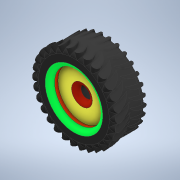
# Autodesk Inventor part: wheel 2
Saved by Autodesk Inventor 2021.3 (Build 253353000, 353)
## iProperties
Created: 2021-07-27
Part Number: wheel 2
Material: Rubber
Document SubType Name: Modeling
Designer: ASUS
Density: 0.93 g/cm^3
Appearance: Rubber - Black
Author: ASUS
Autodesk Inventor part; units mm, degrees
ref_plane "YZ Plane" through (0, 0, 0) normal (1, 0, 0) x (0, 1, 0)
ref_plane "XY Plane" through (0, 0, 0) normal (0, 0, 1) x (1, 0, 0)
sketch "Sketch1" plane through (0, 0, 0) normal (0, 0, 1) x (1, 0, 0)
  circle A0 centre (0, 0) radius 25
  dimension "d0" = 50
  constraints: 1 centre point, 1 coincident
  measures "d0" diameter of A0
extrude "Extrusion1" add sketch "Sketch1" along normal blind 20
fillet "Fillet1" radius 3 2 edges at (-25, 0, 20) (-25, 0, 0)
ref_plane "Work Plane1" through (0, 25, 0) normal (0, 1, 0) x (-1, 0, 0)
sketch "Sketch3" plane through (0, 25, 0) normal (0, 1, 0) x (-1, 0, 0)
  line L0 (25, 3) -> (25, 17) projected
  line L1 (25, 10) -> (-25, 10)
  line L2 (-25, 3) -> (-25, 17) projected
  line L3 (22, 0) -> (-22, 0) projected
  arc A0 (0, 10) -> (-1.7253, 1.0245) centre (24.2725, 0.6808) ccw
  arc A1 (0, 10) -> (-3.7943, 0.9149) centre (6.1349, 2.103) ccw
  arc A2 (-3.7943, 0.9149) -> (-1.7253, 1.0245) centre (-2.7634, 1.0382) ccw
  line L4 (-22, 20) -> (22, 20) projected
  arc A3 (-4.449, 17.997) -> (-2.0455, 10) centre (15.9529, 19.7692) ccw
  arc A4 (-8.7423, 17.2059) -> (-2.0455, 10) centre (1.6814, 20.1783) ccw
  arc A5 (-4.449, 17.997) -> (-8.7423, 17.2059) centre (-6.6336, 17.8072) ccw
  point P0 (0, 0)
  dimension "d5" = 26
  dimension "d6" = 10
  constraints: 16 point on circle, 6 centre point, 6 tangent, 3 midpoint, 2 end point, 1 point on line
  measures "d5" radius of A0
  measures "d6" radius of A1
extrude "Extrusion2" add sketch "Sketch3" against normal blind 5
pattern_circular "Circular Pattern1" count 30 over 360 about axis through (0, 0, 0) along (0, 0, 1) of "Extrusion2"
sketch "Sketch4" plane through (0, 0, 20) normal (0, 0, 1) x (1, 0, 0)
  circle A0 centre (0, 0) radius 17.5
  circle A1 centre (0, 0) radius 3.5
  dimension "d12" = 35
  dimension "d13" = 7
  constraints: 2 centre point, 2 coincident
  measures "d12" diameter of A0
  measures "d13" diameter of A1
extrude "Extrusion3" cut sketch "Sketch4" against normal through all contours A1
sketch "Sketch5" plane through (0, 0, 20) normal (0, 0, 1) x (1, 0, 0)
  circle A0 centre (0, 0) radius 3.5 projected
  circle A1 centre (0, 0) radius 15
  dimension "d16" = 30
  constraints: 1 centre point, 1 coincident
  measures "d16" diameter of A1
extrude "Extrusion4" cut sketch "Sketch5" against normal blind 5
fillet "Fillet2" radius 3 1 edges at (-15, 0, 20)
fillet "Fillet3" radius 3 1 edges at (-3.5, 0, 15)
body "Solid1"
